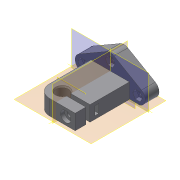
# Autodesk Inventor part: G004162_Cycl_soporteYfrenteIzquierda
Saved by Autodesk Inventor 2015 SP2 (Build 190223200, 223)
## iProperties
Created: 2015-05-04
Part Number: G004162_Cycl_soporteYfrenteIzquierda
Material: Genérico
Document SubType Name: Modeling
Designer: EDU
Density: 1 g/cm^3
Appearance: Valor por defecto
Author: EDU
Autodesk Inventor part; units mm, degrees
sketch "Boceto1" plane through (0, 0, 0) normal (0, 0, 1) x (1, 0, 0)
  line L0 (-13.875, 0) -> (13.875, 0)
  line L1 (13.875, 0) -> (13.875, -39.25)
  line L2 (13.875, -39.25) -> (-13.875, -39.25)
  line L3 (-13.875, -39.25) -> (-13.875, 0)
  point P0 (0, 0)
  point P1 (0, 0)
  dimension "d0" = 27.75
  dimension "d1" = 39.25
  constraints: 8 end point, 2 coincident, 2 parallel, 1 horizontal, 1 midpoint, 1 perpendicular
  measures "d0" distance of L1.end L2.end
  measures "d1" distance of L0.end L1.end
extrude "Extrusión1" add sketch "Boceto1" along normal blind 11
sketch "Boceto3" plane through (0, 0, 0) normal (0, 1, 0) x (-1, 0, 0)
  line L0 (-19.875, 0) -> (19.875, 0)
  line L1 (22.6302, 10.2645) -> (2.7552, 21.7625)
  line L2 (-2.7552, 21.7625) -> (-22.6302, 10.2645)
  line L3 (13.875, 0) -> (-13.875, 0) projected
  arc A0 (-22.6302, 10.2645) -> (-19.875, 0) centre (-19.875, 5.502) ccw
  arc A1 (19.875, 0) -> (22.6302, 10.2645) centre (19.875, 5.502) ccw
  arc A2 (2.7552, 21.7625) -> (-2.7552, 21.7625) centre (0, 17) ccw
  point P0 (0, 0)
  point P1 (0, 23.3564)
  point P2 (0, 0)
  point P3 (0, 0)
  point P4 (0, 0)
  point P5 (0, 0)
  dimension "d21" = 30.05
  dimension "d23" = 39.75
  dimension "d25" = 17
  constraints: 6 end point, 6 point on circle, 6 tangent, 4 midpoint, 3 centre point, 2 equal radius, 2 point on line, 2 vertical alignment, 1 coincident, 1 equal length, 1 horizontal, 1 horizontal alignment
  measures "d21" angle of L0 L1
  measures "d23" distance of A1.centre A0.centre
  measures "d25" distance from line of L0 A2.centre
extrude "Extrusión3" add sketch "Boceto3" along normal blind 10
ref_plane "Plano de trabajo2" through (0, 7.2, 0) normal (0, 1, 0) x (1, 0, 0)
sketch "Boceto5" plane through (0, 7.2, 0) normal (0, 1, 0) x (1, 0, 0)
  line L0 (19.875, 0) -> (-19.875, 0) projected
  arc A0 (-19.875, 0) -> (-22.6302, -10.2645) centre (-19.875, -5.502) ccw projected
  line L1 (-22.6302, -10.2645) -> (-2.7552, -21.7625) projected
  arc A1 (-2.7552, -21.7625) -> (2.7552, -21.7625) centre (0, -17) ccw projected
  line L2 (2.7552, -21.7625) -> (22.6302, -10.2645) projected
  arc A2 (22.6302, -10.2645) -> (19.875, 0) centre (19.875, -5.502) ccw projected
  circle A3 centre (19.875, -5.502) radius 1.875
  circle A4 centre (0, -17) radius 1.875
  circle A5 centre (-19.875, -5.502) radius 1.875
  point P0 (0, 0)
  dimension "d33" = 3.75
  dimension "d34" = 3.75
  dimension "d35" = 3.75
  constraints: 3 centre point, 3 coincident
  measures "d33" diameter of A3
  measures "d34" diameter of A4
  measures "d35" diameter of A5
extrude "Extrusión5" cut sketch "Boceto5" along normal through all both and the other way through all contours A3 | A4 | A5
sketch "Boceto6" plane through (0, 0, 0) normal (0, -1, 0) x (1, 0, 0)
  circle A0 centre (0, 17) radius 1.875 projected
  circle A1 centre (19.875, 5.502) radius 1.875 projected
  circle A2 centre (-19.875, 5.502) radius 1.875 projected
  line L0 (13.875, 0) -> (13.875, 11) projected
  line L1 (19.875, 0) -> (13.875, 0) projected
  arc A3 (19.875, 0) -> (22.6302, 10.2645) centre (19.875, 5.502) ccw projected
  line L2 (2.7552, 21.7625) -> (22.6302, 10.2645) projected
  arc A4 (2.7552, 21.7625) -> (-2.7552, 21.7625) centre (0, 17) ccw projected
  line L3 (-22.6302, 10.2645) -> (-2.7552, 21.7625) projected
  arc A5 (-22.6302, 10.2645) -> (-19.875, 0) centre (-19.875, 5.502) ccw projected
  line L4 (-13.875, 0) -> (-19.875, 0) projected
  line L5 (-13.875, 0) -> (-13.875, 11) projected
  line L6 (13.875, 11) -> (-13.875, 11) projected
  line L7 (-18.0852, 8.602) -> (-16.2954, 5.502)
  line L8 (-16.2954, 5.502) -> (-18.0852, 2.402)
  line L9 (-18.0852, 2.402) -> (-21.6648, 2.402)
  line L10 (-21.6648, 2.402) -> (-23.4546, 5.502)
  line L11 (-23.4546, 5.502) -> (-21.6648, 8.602)
  line L12 (-21.6648, 8.602) -> (-18.0852, 8.602)
  line L13 (1.7898, 20.1) -> (3.5796, 17)
  line L14 (3.5796, 17) -> (1.7898, 13.9)
  line L15 (1.7898, 13.9) -> (-1.7898, 13.9)
  line L16 (-1.7898, 13.9) -> (-3.5796, 17)
  line L17 (-3.5796, 17) -> (-1.7898, 20.1)
  line L18 (-1.7898, 20.1) -> (1.7898, 20.1)
  line L19 (18.0852, 8.602) -> (21.6648, 8.602)
  line L20 (21.6648, 8.602) -> (23.4546, 5.502)
  line L21 (23.4546, 5.502) -> (21.6648, 2.402)
  line L22 (21.6648, 2.402) -> (18.0852, 2.402)
  line L23 (18.0852, 2.402) -> (16.2954, 5.502)
  line L24 (16.2954, 5.502) -> (18.0852, 8.602)
  point P0 (0, 0)
  dimension "d38" = 6.2
  dimension "d39" = 6.2
  dimension "d40" = 6.2
  constraints: 36 end point, 3 coincident, 3 horizontal, 39 other
  measures "d38" distance between parallel lines of L15 L18
  measures "d39" distance between parallel lines of L22 L19
  measures "d40" distance between parallel lines of L9 L12
extrude "Extrusión6" cut sketch "Boceto6" against normal blind 2.8 contours L7 L8 L9 L10 L11 L12 | L13 L14 L15 L16 L17 L18 | L19 L20 L21 L22 L23 L24
ref_plane "Plano de trabajo3" through (-13.875, -23.54, 0) normal (0, -1, 0) x (1, 0, 0)
sketch "Boceto9" plane through (-13.875, -23.54, 0) normal (0, -1, 0) x (1, 0, 0)
  circle A0 centre (6.8, 5.5) radius 1.875 projected
  line L0 (27.75, 11) -> (0, 11) projected
  line L1 (0, 0) -> (0, 11) projected
  line L2 (-21.6528, 0) -> (49.4028, 0) projected
  line L3 (8.7816, 8.5126) -> (10.3998, 5.2902)
  line L4 (10.3998, 5.2902) -> (8.4182, 2.2776)
  line L5 (8.7816, 8.5126) -> (0, 8.5126)
  line L6 (8.4182, 2.2776) -> (0, 2.2776)
  point P0 (13.875, 0)
  dimension "d53" = 120
  dimension "d56" = 6.235
  dimension "d57" = 8.7816
  constraints: 8 end point, 2 perpendicular, 2 point on line, 1 coincident, 4 other
  measures "d53" angle of L4 L3
  measures "d56" distance between parallel lines of L6 L5
  measures "d57" distance of L5.end L3.start
extrude "Extrusión9" cut sketch "Boceto9" along normal mid plane 2.8
sketch "Boceto10" plane through (0, 0, 11) normal (0, 0, 1) x (1, 0, 0)
  line L0 (13.875, -39.25) -> (13.875, 0) projected
  line L1 (-13.875, -39.25) -> (13.875, -39.25) projected
  line L2 (13.875, -28.5) -> (-0.4886, -28.5)
  arc A0 (-0.4886, -28.5) -> (-0.4886, -31.5) centre (-4.625, -30) ccw
  line L3 (-0.4886, -31.5) -> (13.875, -31.5)
  line L4 (-13.875, 0) -> (-13.875, -39.25) projected
  point P0 (0, 0)
  point P1 (-9.025, -30)
  point P2 (-5.7641, -34.25)
  dimension "d60" = 1.5
  dimension "d61" = 5
  dimension "d63" = 7.75
  dimension "d64" = 4.4
  dimension "d89" = 18.5
  constraints: 4 end point, 4 point on circle, 2 point on line, 1 centre point, 1 horizontal, 1 parallel, 1 perpendicular
  measures "d60" distance from line of L3 A0.centre
  measures "d61" distance from line of L1 point (-5.764, -34.25)
  measures "d63" distance between parallel lines of L1 L3
  measures "d64" radius of A0
  measures "d89" distance from line of L0 A0.centre
extrude "Extrusión10" cut sketch "Boceto10" against normal through all
mirror "Simetría1" about plane through (0, 0, 0) normal (1, 0, 0) of "Extrusión9"
sketch "Boceto11" plane through (-13.875, -39.25, 0) normal (-1, 0, 0) x (0, 0, 1)
  line L0 (8.5126, 14.31) -> (2.2776, 14.31) projected
  line L1 (8.5126, 17.11) -> (8.5126, 14.31) projected
  line L2 (2.2776, 17.11) -> (8.5126, 17.11) projected
  line L3 (2.2776, 14.31) -> (2.2776, 17.11) projected
  point P0 (0, 39.25)
extrude "Extrusión11" add sketch "Boceto11" against normal up to surface (13.875 mm away)
sketch "Boceto12" plane through (-13.875, -39.25, 0) normal (0, -1, 0) x (1, 0, 0)
  circle A0 centre (20.95, 5.5) radius 3.75
  line L0 (27.75, 0) -> (0, 0) projected
  line L1 (27.75, 0) -> (27.75, 11) projected
  point P0 (13.875, 0)
  dimension "d69" = 7.5
  dimension "d70" = 5.5
  dimension "d71" = 6.8
  constraints: 1 centre point
  measures "d69" diameter of A0
  measures "d70" distance from line of L0 A0.centre
  measures "d71" distance from line of L1 A0.centre
extrude "Extrusión12" cut sketch "Boceto12" against normal blind 2.8
sketch "Boceto13" plane through (7.075, -36.45, 5.5) normal (0, -1, 0) x (1, 0, 0)
  circle A0 centre (0, 0) radius 3.75 projected
  circle A1 centre (0, 0) radius 1.875
  point P0 (-7.075, -5.5)
  dimension "d74" = 3.75
  constraints: 1 centre point, 1 coincident
  measures "d74" diameter of A1
extrude "Extrusión13" cut sketch "Boceto13" against normal blind 26.4 contours A1
sketch "Boceto14" plane through (0, 0, 0) normal (0, 0, -1) x (-1, 0, 0)
  line L0 (-79.864, -2.1129) -> (-78.9328, -2.1294) construction
  line L1 (-78.9328, -2.1294) -> (-77.7481, -2.2424) construction
  line L2 (-77.7481, -2.2424) -> (-76.5607, -2.4242) construction
  line L3 (-76.5607, -2.4242) -> (-75.3898, -2.6722) construction
  line L4 (-75.3898, -2.6722) -> (-74.2548, -2.9807) construction
  line L5 (-74.3358, -2.9942) -> (-73.2531, -3.3578) construction
  line L6 (-73.2531, -3.3578) -> (-72.242, -3.7683) construction
  line L7 (-72.242, -3.7683) -> (-71.3191, -4.2229) construction
  line L8 (-71.3191, -4.2229) -> (-70.5036, -4.7161) construction
  line L9 (-70.5036, -4.7161) -> (-70.3383, -4.8318) construction
  line L10 (-70.3464, -4.7635) -> (-69.8588, -4.9674) construction
  line L11 (-69.8588, -4.9674) -> (-69.3904, -5.2098) construction
  line L12 (-69.3904, -5.2098) -> (-68.9441, -5.4853) construction
  line L13 (-68.9441, -5.4853) -> (-68.5198, -5.7939) construction
  line L14 (-68.5198, -5.7939) -> (-67.7457, -6.4992) construction
  line L15 (-67.7457, -6.4992) -> (-67.0817, -7.3174) construction
  line L16 (-67.0817, -7.3174) -> (-66.798, -7.761) construction
  line L17 (-66.798, -7.761) -> (-66.5445, -8.2293) construction
  line L18 (-66.5445, -8.2293) -> (-66.3269, -8.717) construction
  line L19 (-66.3269, -8.717) -> (-66.1423, -9.2267) construction
  line L20 (-66.1423, -9.2267) -> (-65.999, -9.7501) construction
  line L21 (-65.999, -9.7501) -> (-65.8834, -10.3584) construction
  line L22 (-65.8834, -10.3584) -> (-65.8614, -10.5512) construction
  line L23 (-65.8614, -10.5512) -> (-70.7846, -10.5512) construction
  line L24 (-70.7846, -10.5512) -> (-70.881, -10.3694) construction
  line L25 (-70.881, -10.3694) -> (-71.1345, -10.0663) construction
  line L26 (-71.1345, -10.0663) -> (-71.4375, -9.8129) construction
  line L27 (-71.4375, -9.8129) -> (-71.7874, -9.6255) construction
  line L28 (-71.7874, -9.6255) -> (-72.1731, -9.5043) construction
  line L29 (-72.1731, -9.5043) -> (-72.5864, -9.463) construction
  line L30 (-72.5864, -9.463) -> (-72.9996, -9.5043) construction
  line L31 (-72.9996, -9.5043) -> (-73.3853, -9.6255) construction
  line L32 (-73.3853, -9.6255) -> (-73.7352, -9.8129) construction
  line L33 (-73.7352, -9.8129) -> (-74.0383, -10.0663) construction
  line L34 (-74.0383, -10.0663) -> (-74.2917, -10.3694) construction
  line L35 (-74.2917, -10.3694) -> (-74.4791, -10.7193) construction
  line L36 (-74.4791, -10.7193) -> (-74.6003, -11.105) construction
  line L37 (-74.6003, -11.105) -> (-74.6416, -11.5182) construction
  line L38 (-74.6416, -11.5182) -> (-74.6003, -11.9315) construction
  line L39 (-74.6003, -11.9315) -> (-74.4791, -12.3172) construction
  line L40 (-74.4791, -12.3172) -> (-74.2917, -12.6671) construction
  line L41 (-74.2917, -12.6671) -> (-74.0383, -12.9701) construction
  line L42 (-74.0383, -12.9701) -> (-73.7352, -13.2209) construction
  line L43 (-73.7352, -13.2209) -> (-73.3853, -13.4109) construction
  line L44 (-73.3853, -13.4109) -> (-72.9996, -13.5294) construction
  line L45 (-72.9996, -13.5294) -> (-72.5864, -13.5707) construction
  line L46 (-72.5864, -13.5707) -> (-72.1731, -13.5294) construction
  line L47 (-72.1731, -13.5294) -> (-71.7874, -13.4109) construction
  line L48 (-71.7874, -13.4109) -> (-71.4375, -13.2209) construction
  line L49 (-71.4375, -13.2209) -> (-71.1345, -12.9701) construction
  line L50 (-71.1345, -12.9701) -> (-70.881, -12.6671) construction
  line L51 (-70.881, -12.6671) -> (-70.6937, -12.3172) construction
  line L52 (-70.6937, -12.3172) -> (-70.6854, -12.2924) construction
  line L53 (-70.6854, -12.2924) -> (-65.8476, -12.2924) construction
  line L54 (-65.8476, -12.2924) -> (-65.9551, -12.9839) construction
  line L55 (-65.9551, -12.9839) -> (-66.1452, -13.6975) construction
  line L56 (-66.1452, -13.6975) -> (-66.4041, -14.378) construction
  line L57 (-66.4041, -14.378) -> (-66.7292, -15.0254) construction
  line L58 (-66.7292, -15.0254) -> (-67.1149, -15.6287) construction
  line L59 (-67.1149, -15.6287) -> (-67.5557, -16.188) construction
  line L60 (-67.5557, -16.188) -> (-68.0489, -16.7004) construction
  line L61 (-68.0489, -16.7004) -> (-68.0379, -16.8327) construction
  line L62 (-68.0379, -16.8327) -> (-67.9772, -17.3561) construction
  line L63 (-67.9772, -17.3561) -> (-67.8726, -17.7914) construction
  line L64 (-67.8726, -17.7914) -> (-67.71, -18.1771) construction
  line L65 (-67.71, -18.1771) -> (-67.4786, -18.5518) construction
  line L66 (-67.4786, -18.5518) -> (-67.1425, -18.9293) construction
  line L67 (-67.1425, -18.9293) -> (-66.7485, -19.2709) construction
  line L68 (-66.7485, -19.2709) -> (-66.0901, -19.6676) construction
  line L69 (-66.0901, -19.6676) -> (-65.3197, -19.9962) construction
  line L70 (-65.3197, -19.9962) -> (-64.4161, -20.2635) construction
  line L71 (-64.4161, -20.2635) -> (-63.3526, -20.4784) construction
  line L72 (-63.3526, -20.4784) -> (-63.1479, -20.5194) construction
  line L73 (-63.1479, -20.5194) -> (-63.1892, -20.5552) construction
  line L74 (-63.1892, -20.5552) -> (-63.8394, -20.7123) construction
  line L75 (-63.8394, -20.7123) -> (-64.6549, -20.8169) construction
  line L76 (-64.6549, -20.8169) -> (-66.4897, -20.8169) construction
  line L77 (-66.4897, -20.8169) -> (-67.6772, -20.704) construction
  line L78 (-67.6772, -20.704) -> (-68.8646, -20.5222) construction
  line L79 (-68.8646, -20.5222) -> (-70.0354, -20.2742) construction
  line L80 (-70.0354, -20.2742) -> (-71.1705, -19.9656) construction
  line L81 (-71.1705, -19.9656) -> (-72.2532, -19.602) construction
  line L82 (-72.2532, -19.602) -> (-73.2643, -19.1915) construction
  line L83 (-73.2643, -19.1915) -> (-74.1872, -18.7369) construction
  line L84 (-74.1872, -18.7369) -> (-75.0027, -18.2438) construction
  line L85 (-75.0027, -18.2438) -> (-75.2011, -18.1005) construction
  line L86 (-75.2011, -18.1005) -> (-75.6805, -17.8911) construction
  line L87 (-75.6805, -17.8911) -> (-76.1433, -17.6487) construction
  line L88 (-76.1433, -17.6487) -> (-77.0001, -17.0618) construction
  line L89 (-77.0001, -17.0618) -> (-77.7605, -16.3566) construction
  line L90 (-77.7605, -16.3566) -> (-78.4134, -15.5438) construction
  line L91 (-78.4134, -15.5438) -> (-78.9424, -14.6347) construction
  line L92 (-78.9424, -14.6347) -> (-79.1573, -14.1498) construction
  line L93 (-79.1573, -14.1498) -> (-79.3364, -13.6456) construction
  line L94 (-79.3364, -13.6456) -> (-79.4796, -13.1277) construction
  line L95 (-79.4796, -13.1277) -> (-79.5816, -12.5904) construction
  line L96 (-79.5816, -12.5904) -> (-79.6449, -12.0422) construction
  line L97 (-79.6449, -12.0422) -> (-79.667, -11.4801) construction
  line L98 (-79.667, -11.4801) -> (-79.6284, -10.7225) construction
  line L99 (-79.6284, -10.7225) -> (-79.5127, -9.9869) construction
  line L100 (-79.5127, -9.9869) -> (-79.3253, -9.2816) construction
  line L101 (-79.3253, -9.2816) -> (-79.0691, -8.6067) construction
  line L102 (-79.0691, -8.6067) -> (-78.7495, -7.9647) construction
  line L103 (-78.7495, -7.9647) -> (-78.3721, -7.3641) construction
  line L104 (-78.3721, -7.3641) -> (-77.9368, -6.8076) construction
  line L105 (-77.9368, -6.8076) -> (-77.4519, -6.2979) construction
  line L106 (-77.4519, -6.2979) -> (-77.4657, -6.1299) construction
  line L107 (-77.4657, -6.1299) -> (-77.5263, -5.6064) construction
  line L108 (-77.5263, -5.6064) -> (-77.6338, -5.1711) construction
  line L109 (-77.6338, -5.1711) -> (-77.7963, -4.7854) construction
  line L110 (-77.7963, -4.7854) -> (-78.0277, -4.4108) construction
  line L111 (-78.0277, -4.4108) -> (-78.3638, -4.0333) construction
  line L112 (-78.3638, -4.0333) -> (-78.8088, -3.6656) construction
  line L113 (-78.8088, -3.6656) -> (-79.4673, -3.2689) construction
  line L114 (-79.4673, -3.2689) -> (-80.1819, -2.9666) construction
  line L115 (-80.1819, -2.9666) -> (-81.0856, -2.6994) construction
  line L116 (-81.0856, -2.6994) -> (-82.149, -2.4845) construction
  line L117 (-82.149, -2.4845) -> (-82.3556, -2.4432) construction
  line L118 (-82.3556, -2.4432) -> (-82.3143, -2.4074) construction
  line L119 (-82.3143, -2.4074) -> (-81.6641, -2.2503) construction
  line L120 (-81.6641, -2.2503) -> (-80.8487, -2.1456) construction
  line L121 (-80.8487, -2.1456) -> (-79.945, -2.1264) construction
  line L122 (-65.8614, -10.5512) -> (-70.7846, -10.5512)
  arc A0 (-70.7846, -10.5512) -> (-70.6854, -12.2924) centre (-72.6298, -11.5297) ccw
  line L123 (-70.6854, -12.2924) -> (-65.8476, -12.2924)
  arc A1 (-68.0489, -16.7004) -> (-65.8476, -12.2924) centre (-72.8859, -11.5313) ccw
  arc A2 (-68.0489, -16.7004) -> (-66.0901, -19.6676) centre (-64.9076, -16.7568) ccw
  arc A3 (-66.0901, -19.6676) -> (-63.1479, -20.5194) centre (-61.5351, -9.4412) ccw
  arc A4 (-75.2011, -18.1005) -> (-63.1479, -20.5194) centre (-65.9638, -3.3112) ccw
  arc A5 (-77.4657, -6.1299) -> (-75.2011, -18.1005) centre (-72.3892, -11.369) ccw
  arc A6 (-77.4657, -6.1299) -> (-79.4673, -3.2689) centre (-80.7471, -6.2949) ccw
  arc A7 (-79.4673, -3.2689) -> (-82.3556, -2.4432) centre (-83.987, -13.6143) ccw
  arc A8 (-70.3464, -4.7635) -> (-82.3556, -2.4432) centre (-79.4561, -19.6741) ccw
  arc A9 (-65.8614, -10.5512) -> (-70.3464, -4.7635) centre (-72.8722, -11.3524) ccw
  line L124 (-50.6216, 1.1163) -> (-50.6216, -28.8837)
  line L125 (-50.6216, 1.1163) -> (-20.6216, 1.1163) construction
  line L126 (-36.3657, -2.4242) -> (-37.5366, -2.6722) construction
  line L127 (-40.6844, -3.7683) -> (-41.6073, -4.2229) construction
  line L128 (-39.6733, -3.3578) -> (-40.6844, -3.7683) construction
  line L129 (-38.5906, -2.9942) -> (-39.6733, -3.3578) construction
  line L130 (-37.5366, -2.6722) -> (-38.6716, -2.9807) construction
  line L131 (-41.6073, -4.2229) -> (-42.4228, -4.7161) construction
  line L132 (-42.4228, -4.7161) -> (-42.5881, -4.8318) construction
  line L133 (-42.58, -4.7635) -> (-43.0676, -4.9674) construction
  line L134 (-43.0676, -4.9674) -> (-43.536, -5.2098) construction
  line L135 (-43.536, -5.2098) -> (-43.9823, -5.4853) construction
  line L136 (-43.9823, -5.4853) -> (-44.4066, -5.7939) construction
  line L137 (-44.4066, -5.7939) -> (-45.1807, -6.4992) construction
  line L138 (-45.1807, -6.4992) -> (-45.8447, -7.3174) construction
  line L139 (-45.8447, -7.3174) -> (-46.1284, -7.761) construction
  line L140 (-46.1284, -7.761) -> (-46.3819, -8.2293) construction
  line L141 (-46.3819, -8.2293) -> (-46.5995, -8.717) construction
  line L142 (-46.5995, -8.717) -> (-46.7841, -9.2267) construction
  line L143 (-46.7841, -9.2267) -> (-46.9274, -9.7501) construction
  line L144 (-46.9274, -9.7501) -> (-47.043, -10.3584) construction
  line L145 (-47.043, -10.3584) -> (-47.065, -10.5512) construction
  line L146 (-42.1418, -10.5512) -> (-42.0454, -10.3694) construction
  line L147 (-40.7533, -9.5043) -> (-40.34, -9.463) construction
  line L148 (-41.139, -9.6255) -> (-40.7533, -9.5043) construction
  line L149 (-41.4889, -9.8129) -> (-41.139, -9.6255) construction
  line L150 (-41.7919, -10.0663) -> (-41.4889, -9.8129) construction
  line L151 (-42.0454, -10.3694) -> (-41.7919, -10.0663) construction
  line L152 (-38.3261, -11.105) -> (-38.2848, -11.5182) construction
  line L153 (-38.2848, -11.5182) -> (-38.3261, -11.9315) construction
  line L154 (-38.3261, -11.9315) -> (-38.4473, -12.3172) construction
  line L155 (-38.4473, -12.3172) -> (-38.6347, -12.6671) construction
  line L156 (-38.4473, -10.7193) -> (-38.3261, -11.105) construction
  line L157 (-38.6347, -12.6671) -> (-38.8881, -12.9701) construction
  line L158 (-38.8881, -12.9701) -> (-39.1912, -13.2209) construction
  line L159 (-39.5411, -13.4109) -> (-39.9268, -13.5294) construction
  line L160 (-39.9268, -13.5294) -> (-40.34, -13.5707) construction
  line L161 (-40.34, -13.5707) -> (-40.7533, -13.5294) construction
  line L162 (-39.1912, -13.2209) -> (-39.5411, -13.4109) construction
  line L163 (-40.7533, -13.5294) -> (-41.139, -13.4109) construction
  line L164 (-41.139, -13.4109) -> (-41.4889, -13.2209) construction
  line L165 (-41.4889, -13.2209) -> (-41.7919, -12.9701) construction
  line L166 (-41.7919, -12.9701) -> (-42.0454, -12.6671) construction
  line L167 (-42.0454, -12.6671) -> (-42.2327, -12.3172) construction
  line L168 (-42.2327, -12.3172) -> (-42.241, -12.2924) construction
  line L169 (-47.0788, -12.2924) -> (-46.9713, -12.9839) construction
  line L170 (-46.9713, -12.9839) -> (-46.7812, -13.6975) construction
  line L171 (-46.7812, -13.6975) -> (-46.5223, -14.378) construction
  line L172 (-46.5223, -14.378) -> (-46.1972, -15.0254) construction
  line L173 (-42.241, -12.2924) -> (-47.0788, -12.2924) construction
  line L174 (-47.065, -10.5512) -> (-42.1418, -10.5512) construction
  line L175 (-46.1972, -15.0254) -> (-45.8115, -15.6287) construction
  line L176 (-45.8115, -15.6287) -> (-45.3707, -16.188) construction
  line L177 (-45.3707, -16.188) -> (-44.8775, -16.7004) construction
  line L178 (-44.8885, -16.8327) -> (-44.9492, -17.3561) construction
  line L179 (-44.9492, -17.3561) -> (-45.0538, -17.7914) construction
  line L180 (-45.0538, -17.7914) -> (-45.2164, -18.1771) construction
  line L181 (-44.8775, -16.7004) -> (-44.8885, -16.8327) construction
  line L182 (-45.2164, -18.1771) -> (-45.4478, -18.5518) construction
  line L183 (-45.4478, -18.5518) -> (-45.7839, -18.9293) construction
  line L184 (-45.7839, -18.9293) -> (-46.1779, -19.2709) construction
  line L185 (-44.0618, -20.5222) -> (-42.891, -20.2742) construction
  line L186 (-45.2492, -20.704) -> (-44.0618, -20.5222) construction
  line L187 (-46.4367, -20.8169) -> (-45.2492, -20.704) construction
  line L188 (-40.34, -9.463) -> (-39.9268, -9.5043) construction
  line L189 (-39.9268, -9.5043) -> (-39.5411, -9.6255) construction
  line L190 (-39.5411, -9.6255) -> (-39.1912, -9.8129) construction
  line L191 (-39.1912, -9.8129) -> (-38.8881, -10.0663) construction
  line L192 (-38.8881, -10.0663) -> (-38.6347, -10.3694) construction
  line L193 (-38.6347, -10.3694) -> (-38.4473, -10.7193) construction
  line L194 (-42.891, -20.2742) -> (-41.7559, -19.9656) construction
  line L195 (-41.7559, -19.9656) -> (-40.6732, -19.602) construction
  line L196 (-40.6732, -19.602) -> (-39.6621, -19.1915) construction
  line L197 (-39.6621, -19.1915) -> (-38.7392, -18.7369) construction
  line L198 (-37.9237, -18.2438) -> (-37.7253, -18.1005) construction
  line L199 (-37.7253, -18.1005) -> (-37.2459, -17.8911) construction
  line L200 (-38.7392, -18.7369) -> (-37.9237, -18.2438) construction
  line L201 (-37.2459, -17.8911) -> (-36.7831, -17.6487) construction
  line L202 (-36.7831, -17.6487) -> (-35.9263, -17.0618) construction
  line L203 (-35.9263, -17.0618) -> (-35.1659, -16.3566) construction
  line L204 (-35.1659, -16.3566) -> (-34.513, -15.5438) construction
  line L205 (-34.513, -15.5438) -> (-33.984, -14.6347) construction
  line L206 (-33.984, -14.6347) -> (-33.7691, -14.1498) construction
  line L207 (-33.7691, -14.1498) -> (-33.59, -13.6456) construction
  line L208 (-33.59, -13.6456) -> (-33.4468, -13.1277) construction
  line L209 (-33.4468, -13.1277) -> (-33.3448, -12.5904) construction
  line L210 (-33.3448, -12.5904) -> (-33.2815, -12.0422) construction
  line L211 (-33.2815, -12.0422) -> (-33.2594, -11.4801) construction
  line L212 (-33.2594, -11.4801) -> (-33.298, -10.7225) construction
  line L213 (-33.298, -10.7225) -> (-33.4137, -9.9869) construction
  line L214 (-33.4137, -9.9869) -> (-33.6011, -9.2816) construction
  line L215 (-33.6011, -9.2816) -> (-33.8573, -8.6067) construction
  line L216 (-33.8573, -8.6067) -> (-34.1769, -7.9647) construction
  line L217 (-34.1769, -7.9647) -> (-34.5543, -7.3641) construction
  line L218 (-34.5543, -7.3641) -> (-34.9896, -6.8076) construction
  line L219 (-33.9936, -2.1294) -> (-35.1783, -2.2424) construction
  line L220 (-35.1783, -2.2424) -> (-36.3657, -2.4242) construction
  line L221 (-34.9896, -6.8076) -> (-35.4745, -6.2979) construction
  line L222 (-35.4745, -6.2979) -> (-35.4607, -6.1299) construction
  line L223 (-35.4607, -6.1299) -> (-35.4001, -5.6064) construction
  line L224 (-35.4001, -5.6064) -> (-35.2926, -5.1711) construction
  line L225 (-35.1301, -4.7854) -> (-34.8987, -4.4108) construction
  line L226 (-34.8987, -4.4108) -> (-34.5626, -4.0333) construction
  line L227 (-34.5626, -4.0333) -> (-34.1176, -3.6656) construction
  line L228 (-35.2926, -5.1711) -> (-35.1301, -4.7854) construction
  line L229 (-33.0624, -2.1129) -> (-33.9936, -2.1294) construction
  line L230 (-34.1176, -3.6656) -> (-33.4591, -3.2689) construction
  line L231 (-33.4591, -3.2689) -> (-32.7445, -2.9666) construction
  line L232 (-32.7445, -2.9666) -> (-31.8408, -2.6994) construction
  line L233 (-32.0777, -2.1456) -> (-32.9814, -2.1264) construction
  line L234 (-46.1779, -19.2709) -> (-46.8363, -19.6676) construction
  line L235 (-46.8363, -19.6676) -> (-47.6067, -19.9962) construction
  line L236 (-48.2715, -20.8169) -> (-46.4367, -20.8169) construction
  line L237 (-47.6067, -19.9962) -> (-48.5103, -20.2635) construction
  line L238 (-49.087, -20.7123) -> (-48.2715, -20.8169) construction
  line L239 (-49.7372, -20.5552) -> (-49.087, -20.7123) construction
  line L240 (-49.7785, -20.5194) -> (-49.7372, -20.5552) construction
  line L241 (-49.5738, -20.4784) -> (-49.7785, -20.5194) construction
  line L242 (-48.5103, -20.2635) -> (-49.5738, -20.4784) construction
  line L243 (-31.2623, -2.2503) -> (-32.0777, -2.1456) construction
  line L244 (-31.8408, -2.6994) -> (-30.7774, -2.4845) construction
  line L245 (-30.7774, -2.4845) -> (-30.5707, -2.4432) construction
  line L246 (-30.6121, -2.4074) -> (-31.2623, -2.2503) construction
  line L247 (-30.5707, -2.4432) -> (-30.6121, -2.4074) construction
  line L248 (-47.065, -10.5512) -> (-42.1418, -10.5512)
  arc A10 (-42.241, -12.2924) -> (-42.1418, -10.5512) centre (-40.2966, -11.5297) ccw
  line L249 (-42.241, -12.2924) -> (-47.0788, -12.2924)
  arc A11 (-47.0788, -12.2924) -> (-44.8775, -16.7004) centre (-40.0405, -11.5313) ccw
  arc A12 (-46.8363, -19.6676) -> (-44.8775, -16.7004) centre (-48.0188, -16.7568) ccw
  arc A13 (-49.7785, -20.5194) -> (-46.8363, -19.6676) centre (-51.3913, -9.4412) ccw
  arc A14 (-49.7785, -20.5194) -> (-37.7253, -18.1005) centre (-46.9626, -3.3112) ccw
  arc A15 (-37.7253, -18.1005) -> (-35.4607, -6.1299) centre (-40.5372, -11.369) ccw
  arc A16 (-33.4591, -3.2689) -> (-35.4607, -6.1299) centre (-32.1793, -6.2949) ccw
  arc A17 (-30.5707, -2.4432) -> (-33.4591, -3.2689) centre (-28.9394, -13.6143) ccw
  arc A18 (-30.5707, -2.4432) -> (-42.58, -4.7635) centre (-33.4703, -19.6741) ccw
  arc A19 (-42.58, -4.7635) -> (-47.065, -10.5512) centre (-40.0542, -11.3524) ccw
  line L250 (-50.6216, -28.8837) -> (-40.6216, -28.8837)
  line L251 (-50.6216, -28.8837) -> (-40.6216, -28.8837) construction
  line L252 (5.0379, -20.669) -> (3.8505, -20.4872) construction
  line L253 (4.8161, -17.305) -> (4.9235, -17.7402) construction
  line L254 (4.9235, -17.7402) -> (5.0861, -18.126) construction
  line L255 (4.7417, -16.6134) -> (4.7555, -16.7815) construction
  line L256 (4.7555, -16.7815) -> (4.8161, -17.305) construction
  line L257 (5.0861, -18.126) -> (5.3175, -18.5006) construction
  line L258 (5.3175, -18.5006) -> (5.6536, -18.8781) construction
  line L259 (6.2225, -20.7819) -> (5.0379, -20.669) construction
  line L260 (5.6536, -18.8781) -> (6.0986, -19.2458) construction
  line L261 (6.0986, -19.2458) -> (6.757, -19.6425) construction
  arc A20 (4.7555, -16.7815) -> (6.757, -19.6425) centre (8.0368, -16.6165) ccw
  line L262 (5.2266, -16.1038) -> (4.7417, -16.6134) construction
  line L263 (6.0393, -14.9466) -> (5.6619, -15.5472) construction
  line L264 (6.3589, -14.3047) -> (6.0393, -14.9466) construction
  line L265 (5.6619, -15.5472) -> (5.2266, -16.1038) construction
  line L266 (-3.3198, -17.7016) -> (-3.7661, -17.4261) construction
  line L267 (-3.7661, -17.4261) -> (-4.1904, -17.1175) construction
  line L268 (-2.8515, -17.944) -> (-3.3198, -17.7016) construction
  line L269 (-2.3638, -18.1479) -> (-2.8515, -17.944) construction
  line L270 (-2.2067, -18.1953) -> (-2.372, -18.0796) construction
  line L271 (-4.1904, -17.1175) -> (-4.9646, -16.4122) construction
  line L272 (-4.9646, -16.4122) -> (-5.6285, -15.594) construction
  line L273 (-5.6285, -15.594) -> (-5.9123, -15.1504) construction
  line L274 (-5.9123, -15.1504) -> (-6.1658, -14.682) construction
  line L275 (-6.1658, -14.682) -> (-6.3834, -14.1944) construction
  line L276 (-6.3834, -14.1944) -> (-6.568, -13.6847) construction
  line L277 (-6.568, -13.6847) -> (-6.7112, -13.1613) construction
  line L278 (-6.7112, -13.1613) -> (-6.8268, -12.553) construction
  line L279 (-6.8268, -12.553) -> (-6.8489, -12.3602) construction
  line L280 (-6.8489, -12.3602) -> (-1.9257, -12.3602) construction
  arc A21 (-6.8489, -12.3602) -> (-2.3638, -18.1479) centre (0.1619, -11.559) ccw
  line L281 (-1.9257, -12.3602) -> (-1.8292, -12.542) construction
  line L282 (-1.8292, -12.542) -> (-1.5758, -12.845) construction
  line L283 (-1.5758, -12.845) -> (-1.2727, -13.0985) construction
  line L284 (-1.2727, -13.0985) -> (-0.9228, -13.2858) construction
  line L285 (-0.9228, -13.2858) -> (-0.5371, -13.4071) construction
  line L286 (-0.5371, -13.4071) -> (-0.1239, -13.4484) construction
  arc A22 (-1.9257, -12.3602) -> (-2.0248, -10.619) centre (-0.0805, -11.3816) ccw
  line L287 (1.7688, -12.1921) -> (1.89, -11.8064) construction
  line L288 (1.89, -11.8064) -> (1.9314, -11.3931) construction
  line L289 (1.9314, -11.3931) -> (1.89, -10.9799) construction
  line L290 (0.2894, -9.382) -> (-0.1239, -9.3406) construction
  line L291 (1.89, -10.9799) -> (1.7688, -10.5942) construction
  line L292 (0.6751, -9.5004) -> (0.2894, -9.382) construction
  line L293 (1.7688, -10.5942) -> (1.5815, -10.2443) construction
  line L294 (1.5815, -10.2443) -> (1.328, -9.9412) construction
  line L295 (1.025, -9.6905) -> (0.6751, -9.5004) construction
  line L296 (1.328, -9.9412) -> (1.025, -9.6905) construction
  line L297 (-2.6748, -2.6372) -> (-1.5397, -2.9457) construction
  arc A23 (2.4908, -4.8109) -> (-9.5623, -2.392) centre (-6.7465, -19.6002) ccw
  line L298 (-3.8457, -2.3892) -> (-2.6748, -2.6372) construction
  line L299 (-4.733, -5.5552) -> (-4.8377, -5.1199) construction
  line L300 (-4.8377, -5.1199) -> (-5.0002, -4.7342) construction
  line L301 (-5.0331, -2.2074) -> (-3.8457, -2.3892) construction
  line L302 (-4.6614, -6.2109) -> (-4.6724, -6.0787) construction
  line L303 (-5.0002, -4.7342) -> (-5.2317, -4.3596) construction
  line L304 (-5.2317, -4.3596) -> (-5.5678, -3.9821) construction
  line L305 (-5.5678, -3.9821) -> (-5.9617, -3.6405) construction
  line L306 (-6.2205, -2.0944) -> (-5.0331, -2.2074) construction
  arc A24 (-4.6614, -6.2109) -> (-6.6202, -3.2438) centre (-7.8027, -6.1546) ccw
  line L307 (-4.6724, -6.0787) -> (-4.733, -5.5552) construction
  line L308 (-6.8626, -10.619) -> (-6.7552, -9.9275) construction
  line L309 (-6.7552, -9.9275) -> (-6.5651, -9.2139) construction
  line L310 (-6.5651, -9.2139) -> (-6.3061, -8.5334) construction
  line L311 (-6.3061, -8.5334) -> (-5.981, -7.886) construction
  line L312 (-2.0248, -10.619) -> (-6.8626, -10.619) construction
  line L313 (-5.981, -7.886) -> (-5.5953, -7.2826) construction
  line L314 (-5.5953, -7.2826) -> (-5.1545, -6.7234) construction
  line L315 (-5.1545, -6.7234) -> (-4.6614, -6.2109) construction
  line L316 (-2.0248, -10.619) -> (-6.8626, -10.619)
  arc A25 (-4.6614, -6.2109) -> (-6.8626, -10.619) centre (0.1756, -11.3801) ccw
  line L317 (-1.5397, -2.9457) -> (-0.457, -3.3094) construction
  line L318 (-0.457, -3.3094) -> (0.5541, -3.7199) construction
  line L319 (0.5541, -3.7199) -> (1.477, -4.1745) construction
  line L320 (2.2925, -4.6676) -> (2.4908, -4.8109) construction
  line L321 (1.477, -4.1745) -> (2.2925, -4.6676) construction
  line L322 (-0.1239, -9.3406) -> (-0.5371, -9.382) construction
  line L323 (-0.9228, -9.5004) -> (-1.2727, -9.6905) construction
  line L324 (-2.0166, -10.5942) -> (-2.0248, -10.619) construction
  line L325 (-1.8292, -10.2443) -> (-2.0166, -10.5942) construction
  line L326 (-1.5758, -9.9412) -> (-1.8292, -10.2443) construction
  line L327 (-1.2727, -9.6905) -> (-1.5758, -9.9412) construction
  line L328 (-0.5371, -9.382) -> (-0.9228, -9.5004) construction
  line L329 (-0.1239, -13.4484) -> (0.2894, -13.4071) construction
  line L330 (0.2894, -13.4071) -> (0.6751, -13.2858) construction
  line L331 (0.6751, -13.2858) -> (1.025, -13.0985) construction
  line L332 (1.025, -13.0985) -> (1.328, -12.845) construction
  line L333 (1.328, -12.845) -> (1.5815, -12.542) construction
  line L334 (1.5815, -12.542) -> (1.7688, -12.1921) construction
  line L335 (-5.9617, -3.6405) -> (-6.6202, -3.2438) construction
  line L336 (-6.6202, -3.2438) -> (-7.3905, -2.9152) construction
  line L337 (-7.3905, -2.9152) -> (-8.2942, -2.6479) construction
  line L338 (-8.0553, -2.0944) -> (-6.2205, -2.0944) construction
  line L339 (-8.2942, -2.6479) -> (-9.3576, -2.433) construction
  line L340 (-8.8708, -2.1991) -> (-8.0553, -2.0944) construction
  line L341 (-9.3576, -2.433) -> (-9.5623, -2.392) construction
  line L342 (-9.5623, -2.392) -> (-9.521, -2.3562) construction
  line L343 (-9.521, -2.3562) -> (-8.8708, -2.1991) construction
  arc A26 (-6.6202, -3.2438) -> (-9.5623, -2.392) centre (-11.1752, -13.4701) ccw
  line L344 (6.2321, -8.2767) -> (6.447, -8.7616) construction
  line L345 (5.7032, -7.3676) -> (6.2321, -8.2767) construction
  line L346 (5.0502, -6.5548) -> (5.7032, -7.3676) construction
  line L347 (4.2899, -5.8495) -> (5.0502, -6.5548) construction
  line L348 (3.4331, -5.2627) -> (4.2899, -5.8495) construction
  line L349 (2.4908, -4.8109) -> (2.9702, -5.0203) construction
  line L350 (2.9702, -5.0203) -> (3.4331, -5.2627) construction
  line L351 (6.447, -8.7616) -> (6.6261, -9.2658) construction
  line L352 (6.6261, -9.2658) -> (6.7694, -9.7837) construction
  line L353 (6.7694, -9.7837) -> (6.8713, -10.321) construction
  arc A27 (4.7555, -16.7815) -> (2.4908, -4.8109) centre (-0.321, -11.5424) ccw
  line L354 (6.8713, -10.321) -> (6.9347, -10.8692) construction
  line L355 (6.9347, -10.8692) -> (6.9567, -11.4312) construction
  line L356 (6.9567, -11.4312) -> (6.9181, -12.1889) construction
  line L357 (6.9181, -12.1889) -> (6.8024, -12.9245) construction
  line L358 (6.8024, -12.9245) -> (6.6151, -13.6297) construction
  line L359 (6.6151, -13.6297) -> (6.3589, -14.3047) construction
  line L360 (6.757, -19.6425) -> (7.4717, -19.9448) construction
  line L361 (7.1537, -20.7985) -> (6.2225, -20.7819) construction
  line L362 (7.4717, -19.9448) -> (8.3753, -20.212) construction
  line L363 (8.1384, -20.7658) -> (7.2348, -20.785) construction
  arc A28 (6.757, -19.6425) -> (9.6454, -20.4682) centre (11.2767, -9.2971) ccw
  line L364 (8.3753, -20.212) -> (9.4388, -20.4269) construction
  line L365 (8.9539, -20.6611) -> (8.1384, -20.7658) construction
  line L366 (9.4388, -20.4269) -> (9.6454, -20.4682) construction
  line L367 (9.6454, -20.4682) -> (9.6041, -20.504) construction
  line L368 (9.6041, -20.504) -> (8.9539, -20.6611) construction
  line L369 (3.8505, -20.4872) -> (2.6796, -20.2392) construction
  arc A29 (-2.3638, -18.1479) -> (9.6454, -20.4682) centre (6.7458, -3.2373) ccw
  line L370 (2.6796, -20.2392) -> (1.5445, -19.9306) construction
  line L371 (1.6255, -19.9172) -> (0.5428, -19.5535) construction
  line L372 (0.5428, -19.5535) -> (-0.4683, -19.143) construction
  line L373 (-0.4683, -19.143) -> (-1.3912, -18.6885) construction
  line L374 (-1.3912, -18.6885) -> (-2.2067, -18.1953) construction
  line L375 (-6.8489, -12.3602) -> (-1.9257, -12.3602)
  point P0 (0, 0)
  dimension "d80" = 30
  dimension "d81" = 90
  dimension "d84" = 10
  dimension "d85" = 0
  constraints: 752 end point, 72 point on circle, 30 centre point, 7 tangent, 3 horizontal, 2 collinear, 2 equal length, 1 vertical
  measures "d80" distance of L124.start L124.end
  measures "d81" angle of L124 L125
  measures "d84" distance of L124.end L250.end
  measures "d85" distance between parallel lines of L250 L251
extrude "Extrusión16" cut sketch "Boceto14" against normal blind 2 contours A20 A28 A29 A21 L375 A22 L316 A25 A24 A26 A23 A27
fillet "Empalme3" radius 9.25 1 edges at (-13.875, -39.25, 5.5)
chamfer "Chamfer1" distance 1 angle 30 2 edges at (-9.025, -30, 11) (-9.025, -30, 0) measured on face at (-0.7846, -27.8526, 3.6667)
